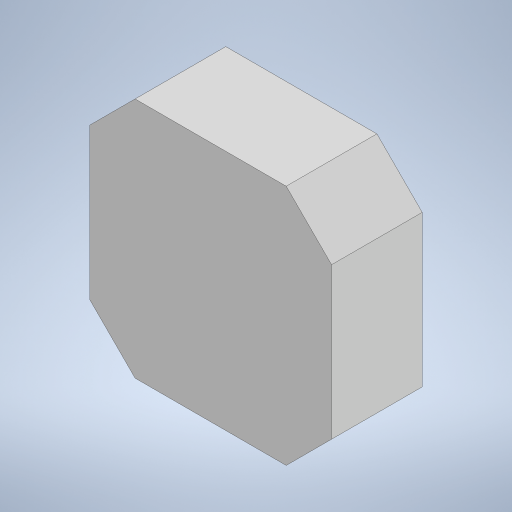
# Autodesk Inventor part: Steckdosen_Block
Saved by Autodesk Inventor 2024 (Build 280153000, 153)
## iProperties
Created: 2026-06-01
Part Number: Steckdosen_Block
Material: Generisch
Document SubType Name: Modeling
Designer: maxim
Density: 1 g/cm^3
Appearance: Vorgabe
Author: maxim
Autodesk Inventor part; units mm, degrees
ref_plane "YZ Plane" through (0, 0, 0) normal (1, 0, 0) x (0, 1, 0)
ref_plane "XZ Plane" through (0, 0, 0) normal (0, 1, 0) x (-1, 0, 0)
ref_plane "XY Plane" through (0, 0, 0) normal (0, 0, 1) x (1, 0, 0)
sketch "Skizze1" plane through (0, 0, 0) normal (0, 1, 0) x (-1, 0, 0)
  line L0 (0, 0) -> (32, 0)
  line L1 (32, 0) -> (32, -32)
  line L2 (32, -32) -> (0, -32)
  line L3 (0, -32) -> (0, 0)
  dimension "d0" = 32
  dimension "d1" = 32
  constraints: 8 end point, 2 parallel, 1 horizontal, 1 perpendicular
  measures "d0" distance of L1.end L2.end
  measures "d1" distance of L0.end L1.end
extrude "Extrusion1" add sketch "Skizze1" along normal blind 12
sketch "Skizze2" plane through (0, 12, 0) normal (0, 1, 0) x (1, 0, 0)
  circle A0 centre (-24, 8) radius 2.2
  line L0 (-32, 32) -> (-32, 0) projected
  line L1 (-32, 0) -> (0, 0) projected
  circle A1 centre (-24, 24) radius 2.2
  circle A2 centre (-8, 8) radius 2.2
  circle A3 centre (-8, 24) radius 2.2
  dimension "d4" = 4.4
  dimension "d6" = 8
  dimension "d7" = 8
  dimension "d10" = 16
  dimension "d13" = 16
  constraints: 4 centre point, 1 horizontal, 1 vertical, 6 other
  measures "d4" diameter of A0
  measures "d6" distance from line of L1 A0.centre
  measures "d7" distance from line of A0.centre L0
  measures "d10" distance of A0.centre A1.centre
  measures "d13" distance of A0.centre A2.centre
extrude "Extrusion2" cut sketch "Skizze2" against normal blind 6
chamfer "Fasen1" distance 6 angle 45 4 edges at (0, 6, 0) (-32, 6, 0) (-32, 6, -32) (0, 6, -32)
